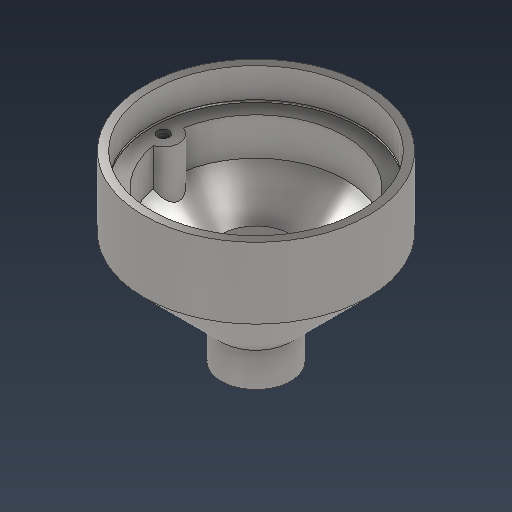
# Autodesk Inventor part: 18102021-002-08
Saved by Autodesk Inventor 2021 (Build 250183000, 183)
## iProperties
Created: 2021-10-17
Part Number: 18102021-002-08
Material: Stainless Steel
Document SubType Name: Modeling
Designer: DuctopwH
Density: 8 g/cm^3
Appearance: Semi-Polished
Author: DuctopwH
Autodesk Inventor part; units mm, degrees
ref_plane "YZ Plane" through (0, 0, 0) normal (1, 0, 0) x (0, 1, 0)
ref_plane "XZ Plane" through (0, 0, 0) normal (0, 1, 0) x (-1, 0, 0)
sketch "Sketch1" plane through (0, 0, 0) normal (0, 0, 1) x (1, 0, 0)
  line L0 (0, 0) -> (0, 8)
  line L1 (-3.5, 0) -> (-3.5, 16)
  line L2 (-3.5, 16) -> (-6, 16)
  line L3 (-6, 16) -> (-6, 10.1213)
  line L4 (-6, 10.1213) -> (-15.3787, 19.5)
  line L5 (-3.5, 0) -> (-6, 0)
  line L6 (-6, 0) -> (-6, 5.8787)
  line L7 (-6, 5.8787) -> (-19.3813, 19.26)
  line L8 (-19.3813, 19.26) -> (-19.3813, 31.5)
  line L9 (-19.3813, 31.5) -> (-18, 31.5)
  line L10 (-6, 10.1213) -> (-6, 5.8787)
  line L11 (-6, 8) -> (0, 8)
  line L12 (-15.3787, 19.5) -> (-15.3787, 26)
  line L13 (-15.3787, 26) -> (-18, 26)
  line L14 (-18, 26) -> (-18, 31.5)
  dimension "d0" = 7
  dimension "d1" = 12
  dimension "d2" = 45
  dimension "d3" = 16
  dimension "d5" = 12.24
  dimension "d6" = 3
  dimension "d7" = 31.5
  dimension "d8" = 8
  dimension "d28" = 36
  dimension "d29" = 12
  dimension "d30" = 6.5
  constraints: 30 end point, 6 perpendicular, 4 vertical, 2 horizontal, 2 parallel, 1 collinear, 1 midpoint, 1 point on line
  measures "d0" diameter of L1 L0
  measures "d1" diameter of L6 L0
  measures "d2" angle of L0 L4
  measures "d3" distance between parallel lines of L5 L2
  measures "d5" distance from line of L7.end L9
  measures "d6" distance between parallel lines of L7 L4
  measures "d7" distance between parallel lines of L5 L9
  measures "d8" distance of L0.start L0.end
  measures "d28" diameter of L14 L0
  measures "d29" distance from line of L9 L4.end
  measures "d30" distance from line of L4.end L13
revolve "Revolution1" add sketch "Sketch1" angle 360 about axis through (0, 0, 0) along (0, 1, 0)
ref_plane "Work Plane1" through (0, 26, 0) normal (0, 1, 0) x (1, 0, 0)
sketch "Sketch2" plane through (0, 26, 0) normal (0, 1, 0) x (1, 0, 0)
  circle A0 centre (-16, 0) radius 2.75
  line L0 (0, 0) -> (0, 15.3787)
  circle A1 centre (0, 0) radius 15.3787 projected
  circle A2 centre (16, 0) radius 2.75
  point P0 (15.1544, 2.6168)
  point P1 (15.1544, -2.6168)
  point P2 (-15.1544, 2.6168)
  point P3 (-15.1544, -2.6168)
  point P4 (-15.1544, 2.6168)
  point P5 (-15.1544, -2.6168)
  dimension "d11" = 32
  dimension "d12" = 5.5
  dimension "d35" = 5.2335
  constraints: 5 point on circle, 2 centre point, 2 end point, 1 horizontal alignment, 1 symmetric about line, 1 vertical, 1 other
  measures "d11" distance of A2.centre A0.centre
  measures "d12" diameter of A0
  measures "d35" distance of A0.end A0.start
extrude "Extrusion1" add sketch "Sketch2" against normal up to surface contours A0 A1 | A2 A1 picked at (-14.6525, 0) picked at (14.7143, -0.6004)
sketch "Sketch3" plane through (0, 26, 0) normal (0, 1, 0) x (1, 0, 0)
  arc A0 (-15.1544, -2.6168) -> (-15.1544, 2.6168) centre (-16, 0) ccw projected
  arc A1 (15.1544, 2.6168) -> (15.1544, -2.6168) centre (16, 0) ccw projected
  point P0 (0, 0)
  point P1 (-17.8887, -1.9989)
  point P2 (-17.8887, 1.9989)
  point P3 (17.8887, 1.9989)
  point P4 (17.8887, -1.9989)
  constraints: 2 coincident
sketch "Sketch4" plane through (0, 0, 0) normal (0, 0, 1) x (1, 0, 0)
  circle A0 centre (-18, 26.2) radius 0.2
  line L0 (0, 25.76) -> (0, 31.5)
  line L1 (18, 26) -> (-18, 26) projected
  line L2 (-18, 31.5) -> (-18, 26) projected
  point P0 (0, 0)
  point P1 (-15.1544, 26)
  dimension "d15" = 0.4
  constraints: 2 end point, 1 point on line, 1 vertical alignment, 2 other
revolve "Revolution2" cut sketch "Sketch4" angle 360 about axis through (0, 25.76, 0) along (0, 1, 0)
hole "Hole1" at (-16, 26, 0) at (16, 26, 0) direction (0, -1, 0) diameter 2.013 depth 7 tip angle 118 thread size "M2.5x0.45" class "6H" standard "ANSI Metric M Profile"
sketch "Sketch7" plane through (0, 31.5, 0) normal (0, 1, 0) x (1, 0, 0)
  line L0 (31.4446, -31.0263) -> (0, -31.0263)
  line L1 (0, -31.0263) -> (0, 28.9425)
  line L2 (0, 28.9425) -> (31.4446, 28.9425)
  line L3 (31.4446, 28.9425) -> (31.4446, -31.0263)
  point P0 (0, 0)
  constraints: 8 end point, 2 parallel, 1 horizontal, 1 perpendicular
body "Solid1"
